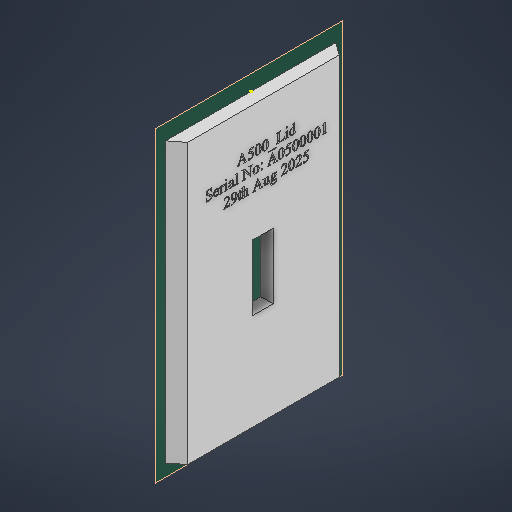
# Autodesk Inventor part: A500_Lid
Saved by Autodesk Inventor 2026.1 (Build 301233000, 233)
## iProperties
Created: 2025-08-29
Part Number: A500_Lid
Material: Generic
Document SubType Name: Modeling
Designer: usman
Density: 1 g/cm^3
Appearance: Default
Author: usman
Autodesk Inventor part; units mm, degrees
(part 1 of 2)
ref_plane "YZ Plane" through (0, 0, 0) normal (1, 0, 0) x (0, 1, 0)
ref_plane "XZ Plane" through (0, 0, 0) normal (0, 1, 0) x (-1, 0, 0)
ref_plane "XY Plane" through (0, 0, 0) normal (0, 0, 1) x (1, 0, 0)
sketch "Sketch1" plane through (0, 0, 0) normal (1, 0, 0) x (0, 1, 0)
  line L0 (-89.45, 54.5) -> (89.45, 54.5)
  line L1 (89.45, 54.5) -> (89.45, -54.5)
  line L2 (89.45, -54.5) -> (-89.45, -54.5)
  line L3 (-89.45, -54.5) -> (-89.45, 54.5)
  line L4 (-89.45, 54.5) -> (89.45, -54.5) construction
  line L5 (89.45, 54.5) -> (-89.45, -54.5) construction
  point P0 (0, 0)
  dimension "d0" = 178.9
  dimension "d1" = 109
  constraints: 12 end point, 2 midpoint, 2 parallel, 1 horizontal, 1 perpendicular
  measures "d0" distance of L0.start L0.end
  measures "d1" distance of L0.end L1.end
extrude "Extrusion1" add sketch "Sketch1" along normal blind 8
sketch "Sketch2" plane through (0, 89.45, 54.5) normal (0, 1, 0) x (1, 0, 0)
  point P0 (0, 54.5)
sketch "Sketch3" plane through (0, 89.45, 54.5) normal (0, 1, 0) x (1, 0, 0)
  line L0 (0, 0) -> (8, 0) projected
  line L1 (0, 0) -> (8, 6.2837)
  line L2 (8, 109) -> (8, 0) projected
  line L3 (0, 109) -> (8, 109) projected
  line L4 (0, 109) -> (8, 103.3983)
  line L5 (0, 109) -> (0, 0) projected
  line L6 (0, 0) -> (8, 0)
  line L7 (0, 109) -> (8, 109)
  line L8 (8, 103.3983) -> (8, 109)
  point P0 (0, 54.5)
  dimension "d4" = 125
  constraints: 10 end point, 3 collinear, 2 point on line
  measures "d4" angle of L5 L4
extrude "Extrusion2" cut sketch "Sketch3" against normal through all contours L1 L2 L0 | L3 L2 L4
sketch "Sketch4" plane through (8, 0, 0) normal (1, 0, 0) x (0, 0, -1)
  line L0 (6.5, 14.45) -> (-6.5, 14.45)
  line L1 (-6.5, 14.45) -> (-6.5, -27.55)
  line L2 (-6.5, -27.55) -> (6.5, -27.55)
  line L3 (6.5, -27.55) -> (6.5, 14.45)
  line L4 (6.5, 14.45) -> (-6.5, -27.55) construction
  line L5 (-6.5, 14.45) -> (6.5, -27.55) construction
  line L6 (48.8983, 89.45) -> (-48.2163, 89.45) projected
  line L7 (-54.5, 89.45) -> (-54.5, -89.45) projected
  point P0 (0, 0)
  point P1 (0, -6.55)
  dimension "d7" = 75
  dimension "d8" = 42
  dimension "d9" = 13
  dimension "d10" = 54.5
  constraints: 12 end point, 2 midpoint, 2 parallel, 1 horizontal, 1 perpendicular
  measures "d7" distance between parallel lines of L0 L6
  measures "d8" distance of L0.end L1.end
  measures "d9" distance of L1.end L2.end
  measures "d10" distance from line of L7 point (0, -6.55)
extrude "Extrusion3" cut sketch "Sketch4" against normal through all
sketch "Sketch6" plane through (8, 0, 0) normal (1, 0, 0) x (0, 0, -1)
  line L0 (-41.7469, 84.5581) -> (46.2409, 84.5581) construction
  line L1 (46.2409, 84.5581) -> (46.2409, 20.4595) construction
  line L2 (46.2409, 20.4595) -> (-41.7469, 20.4595) construction
  line L3 (-41.7469, 20.4595) -> (-41.7469, 84.5581) construction
  line L4 (-12.4626, 61.9812) -> (-14.8333, 61.9812)
  line L5 (-14.8333, 61.9812) -> (-15.2466, 61.025)
  spline S0 degree 2 poles (-15.2466, 61.025) (-15.401, 60.6664) (-15.401, 60.4921) knots 0 0 0 1 1 1
  spline S1 degree 2 poles (-15.401, 60.4921) (-15.401, 60.3526) (-15.1321, 60.1385) (-14.6938, 60.1086) knots 0 0 0 1 2 2 2
  line L6 (-14.6938, 60.1086) -> (-14.6938, 59.9442)
  line L7 (-14.6938, 59.9442) -> (-16.6162, 59.9442)
  line L8 (-16.6162, 59.9442) -> (-16.6162, 60.1086)
  spline S2 degree 2 poles (-16.6162, 60.1086) (-16.2327, 60.1783) (-16.1232, 60.2829) knots 0 0 0 1 1 1
  spline S3 degree 2 poles (-16.1232, 60.2829) (-15.8941, 60.502) (-15.6152, 61.1644) knots 0 0 0 1 1 1
  line L9 (-15.6152, 61.1644) -> (-13.4636, 66.1797)
  line L10 (-13.4636, 66.1797) -> (-13.3043, 66.1797)
  line L11 (-13.3043, 66.1797) -> (-11.1826, 61.1096)
  spline S4 degree 2 poles (-11.1826, 61.1096) (-10.9286, 60.497) (-10.5103, 60.1335) (-10.1367, 60.1086) knots 0 0 0 1 2 2 2
  line L12 (-10.1367, 60.1086) -> (-10.1367, 59.9442)
  line L13 (-10.1367, 59.9442) -> (-12.5423, 59.9442)
  line L14 (-12.5423, 59.9442) -> (-12.5423, 60.1086)
  spline S5 degree 2 poles (-12.5423, 60.1086) (-12.1787, 60.1285) (-11.9197, 60.3327) (-11.9197, 60.4821) knots 0 0 0 1 2 2 2
  spline S6 degree 2 poles (-11.9197, 60.4821) (-11.9197, 60.6813) (-12.099, 61.1096) knots 0 0 0 1 1 1
  line L15 (-12.099, 61.1096) -> (-12.4626, 61.9812)
  line L16 (-12.602, 62.3149) -> (-13.628, 64.7802)
  line L17 (-13.628, 64.7802) -> (-14.6938, 62.3149)
  line L18 (-14.6938, 62.3149) -> (-12.602, 62.3149)
  line L19 (-6.0379, 66.0402) -> (-6.3865, 65.2782)
  line L20 (-6.3865, 65.2782) -> (-8.2193, 65.2782)
  line L21 (-8.2193, 65.2782) -> (-8.6227, 64.4614)
  spline S7 degree 2 poles (-8.6227, 64.4614) (-7.4324, 64.2871) (-6.7351, 63.5749) knots 0 0 0 1 1 1
  spline S8 degree 2 poles (-6.7351, 63.5749) (-6.1375, 62.9623) (-6.1375, 62.1356) knots 0 0 0 1 1 1
  spline S9 degree 2 poles (-6.1375, 62.1356) (-6.1375, 61.6575) (-6.5309, 60.8357) (-7.1236, 60.263) (-7.4872, 60.0886) knots 0 0 0 1 2 3 3 3
  spline S10 degree 2 poles (-7.4872, 60.0886) (-8.0051, 59.8396) (-8.548, 59.8396) knots 0 0 0 1 1 1
  spline S11 degree 2 poles (-8.548, 59.8396) (-9.1008, 59.8396) (-9.5989, 60.2132) (-9.5989, 60.4373) knots 0 0 0 1 2 2 2
  spline S12 degree 2 poles (-9.5989, 60.4373) (-9.5989, 60.5618) (-9.3947, 60.756) (-9.2353, 60.756) knots 0 0 0 1 2 2 2
  spline S13 degree 2 poles (-9.2353, 60.756) (-9.1207, 60.756) (-8.9415, 60.6813) (-8.7323, 60.5319) knots 0 0 0 1 2 2 2
  spline S14 degree 2 poles (-8.7323, 60.5319) (-8.3936, 60.3028) (-8.045, 60.2978) knots 0 0 0 1 1 1
  spline S15 degree 2 poles (-8.045, 60.2978) (-7.522, 60.2978) (-6.7202, 61.0947) (-6.7202, 61.6674) knots 0 0 0 1 2 2 2
  spline S16 degree 2 poles (-6.7202, 61.6674) (-6.7202, 62.2203) (-7.4324, 63.1815) (-8.0599, 63.4405) knots 0 0 0 1 2 2 2
  spline S17 degree 2 poles (-8.0599, 63.4405) (-8.548, 63.6446) (-9.3947, 63.6745) knots 0 0 0 1 1 1
  line L22 (-9.3947, 63.6745) -> (-8.2243, 66.0402)
  line L23 (-8.2243, 66.0402) -> (-6.0379, 66.0402)
  spline S18 degree 2 poles (-5.0966, 62.9574) (-5.0966, 63.9983) (-4.4691, 65.5023) (-3.9461, 65.8709) knots 0 0 0 1 2 2 2
  spline S19 degree 2 poles (-3.9461, 65.8709) (-3.5427, 66.1647) (-3.1094, 66.1647) knots 0 0 0 1 1 1
  spline S20 degree 2 poles (-3.1094, 66.1647) (-2.4072, 66.1647) (-1.8494, 65.4525) knots 0 0 0 1 1 1
  spline S21 degree 2 poles (-1.8494, 65.4525) (-1.1521, 64.566) (-1.1521, 63.052) knots 0 0 0 1 1 1
  spline S22 degree 2 poles (-1.1521, 63.052) (-1.1521, 61.9912) (-1.7647, 60.507) (-2.711, 59.8396) (-3.1542, 59.8396) knots 0 0 0 1 2 3 3 3
  spline S23 degree 2 poles (-3.1542, 59.8396) (-4.0258, 59.8396) (-4.6085, 60.8706) knots 0 0 0 1 1 1
  spline S24 degree 2 poles (-4.6085, 60.8706) (-5.0966, 61.7372) (-5.0966, 62.9574) knots 0 0 0 1 1 1
  spline S25 degree 2 poles (-4.2151, 62.8428) (-4.2151, 61.5877) (-3.9063, 60.7909) knots 0 0 0 1 1 1
  spline S26 degree 2 poles (-3.9063, 60.7909) (-3.6473, 60.1235) (-3.1393, 60.1235) knots 0 0 0 1 1 1
  spline S27 degree 2 poles (-3.1393, 60.1235) (-2.8953, 60.1235) (-2.3773, 60.5568) (-2.2428, 61.0698) knots 0 0 0 1 2 2 2
  spline S28 degree 2 poles (-2.2428, 61.0698) (-2.0336, 61.8417) (-2.0336, 63.2462) knots 0 0 0 1 1 1
  spline S29 degree 2 poles (-2.0336, 63.2462) (-2.0336, 64.2921) (-2.2478, 64.9844) knots 0 0 0 1 1 1
  spline S30 degree 2 poles (-2.2478, 64.9844) (-2.4122, 65.5023) (-2.6662, 65.7165) knots 0 0 0 1 1 1
  spline S31 degree 2 poles (-2.6662, 65.7165) (-2.8504, 65.8659) (-3.1144, 65.8659) knots 0 0 0 1 1 1
  spline S32 degree 2 poles (-3.1144, 65.8659) (-3.4182, 65.8659) (-3.6573, 65.592) knots 0 0 0 1 1 1
  spline S33 degree 2 poles (-3.6573, 65.592) (-3.981, 65.2185) (-4.2151, 63.6197) (-4.2151, 62.8428) knots 0 0 0 1 2 2 2
  spline S34 degree 2 poles (-0.4897, 62.9574) (-0.4897, 63.9983) (0.1378, 65.5023) (0.6607, 65.8709) knots 0 0 0 1 2 2 2
  spline S35 degree 2 poles (0.6607, 65.8709) (1.0642, 66.1647) (1.4975, 66.1647) knots 0 0 0 1 1 1
  spline S36 degree 2 poles (1.4975, 66.1647) (2.1997, 66.1647) (2.7575, 65.4525) knots 0 0 0 1 1 1
  spline S37 degree 2 poles (2.7575, 65.4525) (3.4547, 64.566) (3.4547, 63.052) knots 0 0 0 1 1 1
  spline S38 degree 2 poles (3.4547, 63.052) (3.4547, 61.9912) (2.8422, 60.507) (1.8959, 59.8396) (1.4526, 59.8396) knots 0 0 0 1 2 3 3 3
  spline S39 degree 2 poles (1.4526, 59.8396) (0.5811, 59.8396) (-0.0016, 60.8706) knots 0 0 0 1 1 1
  spline S40 degree 2 poles (-0.0016, 60.8706) (-0.4897, 61.7372) (-0.4897, 62.9574) knots 0 0 0 1 1 1
  spline S41 degree 2 poles (0.3918, 62.8428) (0.3918, 61.5877) (0.7006, 60.7909) knots 0 0 0 1 1 1
  spline S42 degree 2 poles (0.7006, 60.7909) (0.9596, 60.1235) (1.4676, 60.1235) knots 0 0 0 1 1 1
  spline S43 degree 2 poles (1.4676, 60.1235) (1.7116, 60.1235) (2.2296, 60.5568) (2.364, 61.0698) knots 0 0 0 1 2 2 2
  spline S44 degree 2 poles (2.364, 61.0698) (2.5732, 61.8417) (2.5732, 63.2462) knots 0 0 0 1 1 1
  spline S45 degree 2 poles (2.5732, 63.2462) (2.5732, 64.2921) (2.3591, 64.9844) knots 0 0 0 1 1 1
  spline S46 degree 2 poles (2.3591, 64.9844) (2.1947, 65.5023) (1.9407, 65.7165) knots 0 0 0 1 1 1
  spline S47 degree 2 poles (1.9407, 65.7165) (1.7564, 65.8659) (1.4925, 65.8659) knots 0 0 0 1 1 1
  spline S48 degree 2 poles (1.4925, 65.8659) (1.1887, 65.8659) (0.9496, 65.592) knots 0 0 0 1 1 1
  spline S49 degree 2 poles (0.9496, 65.592) (0.6259, 65.2185) (0.3918, 63.6197) (0.3918, 62.8428) knots 0 0 0 1 2 2 2
  line L24 (8.47, 57.962) -> (3.7087, 57.962)
  line L25 (3.7087, 57.962) -> (3.7087, 58.3405)
  line L26 (3.7087, 58.3405) -> (8.47, 58.3405)
  line L27 (8.47, 58.3405) -> (8.47, 57.962)
  line L28 (13.6695, 61.6326) -> (13.8189, 61.6027)
  line L29 (13.8189, 61.6027) -> (13.296, 59.9442)
  line L30 (13.296, 59.9442) -> (8.5796, 59.9442)
  line L31 (8.5796, 59.9442) -> (8.5796, 60.1086)
  line L32 (8.5796, 60.1086) -> (8.8087, 60.1086)
  spline S50 degree 2 poles (8.8087, 60.1086) (9.1922, 60.1086) (9.3565, 60.3626) knots 0 0 0 1 1 1
  spline S51 degree 2 poles (9.3565, 60.3626) (9.4511, 60.502) (9.4511, 61.025) knots 0 0 0 1 1 1
  line L33 (9.4511, 61.025) -> (9.4511, 64.9595)
  spline S52 degree 2 poles (9.4511, 64.9595) (9.4511, 65.5322) (9.3266, 65.6766) knots 0 0 0 1 1 1
  spline S53 degree 2 poles (9.3266, 65.6766) (9.1523, 65.8759) (8.8087, 65.8759) knots 0 0 0 1 1 1
  line L34 (8.8087, 65.8759) -> (8.5796, 65.8759)
  line L35 (8.5796, 65.8759) -> (8.5796, 66.0402)
  line L36 (8.5796, 66.0402) -> (11.3337, 66.0402)
  line L37 (11.3337, 66.0402) -> (11.3337, 65.8759)
  spline S54 degree 2 poles (11.3337, 65.8759) (10.8456, 65.8808) (10.4572, 65.6916) (10.3127, 65.4027) (10.3127, 64.8599) knots 0 0 0 1 2 3 3 3
  line L38 (10.3127, 64.8599) -> (10.3127, 61.0299)
  spline S55 degree 2 poles (10.3127, 61.0299) (10.3127, 60.6564) (10.3825, 60.517) knots 0 0 0 1 1 1
  spline S56 degree 2 poles (10.3825, 60.517) (10.4373, 60.4223) (10.6614, 60.3327) (11.254, 60.3327) knots 0 0 0 1 2 2 2
  line L39 (11.254, 60.3327) -> (11.6973, 60.3327)
  spline S57 degree 2 poles (11.6973, 60.3327) (12.3995, 60.3327) (12.9673, 60.5419) (13.4355, 61.0648) (13.6695, 61.6326) knots 0 0 0 1 2 3 3 3
  line L40 (15.7215, 64.1825) -> (15.7215, 60.8755)
  spline S58 degree 2 poles (15.7215, 60.8755) (15.7215, 60.4921) (15.831, 60.2331) (16.0551, 60.1086) (16.344, 60.1086) knots 0 0 0 1 2 3 3 3
  line L41 (16.344, 60.1086) -> (16.344, 59.9442)
  line L42 (16.344, 59.9442) -> (14.3469, 59.9442)
  line L43 (14.3469, 59.9442) -> (14.3469, 60.1086)
  spline S59 degree 2 poles (14.3469, 60.1086) (14.6457, 60.1086) (14.8549, 60.2231) (14.9744, 60.4921) (14.9744, 60.8755) knots 0 0 0 1 2 3 3 3
  line L44 (14.9744, 60.8755) -> (14.9744, 62.4593)
  spline S60 degree 2 poles (14.9744, 62.4593) (14.9744, 63.1267) (14.9345, 63.3259) knots 0 0 0 1 1 1
  spline S61 degree 2 poles (14.9345, 63.3259) (14.9047, 63.4703) (14.7652, 63.5849) (14.6507, 63.5849) knots 0 0 0 1 2 2 2
  spline S62 degree 2 poles (14.6507, 63.5849) (14.5262, 63.5849) (14.3469, 63.5152) knots 0 0 0 1 1 1
  line L45 (14.3469, 63.5152) -> (14.2821, 63.6795)
  line L46 (14.2821, 63.6795) -> (15.5222, 64.1825)
  line L47 (15.5222, 64.1825) -> (15.7215, 64.1825)
  spline S63 degree 2 poles (15.3479, 66.339) (15.5372, 66.339) (15.8011, 66.0751) (15.8011, 65.8858) knots 0 0 0 1 2 2 2
  spline S64 degree 2 poles (15.8011, 65.8858) (15.8011, 65.6966) (15.5372, 65.4276) (15.3479, 65.4276) knots 0 0 0 1 2 2 2
  spline S65 degree 2 poles (15.3479, 65.4276) (15.1587, 65.4276) (14.8897, 65.6966) (14.8897, 65.8858) knots 0 0 0 1 2 2 2
  spline S66 degree 2 poles (14.8897, 65.8858) (14.8897, 66.0751) (15.1537, 66.339) (15.3479, 66.339) knots 0 0 0 1 2 2 2
  spline S67 degree 2 poles (19.7655, 60.4074) (19.4667, 60.0936) (18.889, 59.8197) (18.5553, 59.8197) knots 0 0 0 1 2 2 2
  spline S68 degree 2 poles (18.5553, 59.8197) (17.8829, 59.8197) (16.8769, 60.9453) (16.8769, 61.8318) knots 0 0 0 1 2 2 2
  spline S69 degree 2 poles (16.8769, 61.8318) (16.8769, 62.7133) (17.9925, 64.1825) (18.8691, 64.1825) knots 0 0 0 1 2 2 2
  spline S70 degree 2 poles (18.8691, 64.1825) (19.4119, 64.1825) (19.7655, 63.8339) knots 0 0 0 1 1 1
  line L48 (19.7655, 63.8339) -> (19.7655, 64.6059)
  spline S71 degree 2 poles (19.7655, 64.6059) (19.7655, 65.3081) (19.6958, 65.6268) (19.5564, 65.7414) (19.4468, 65.7414) knots 0 0 0 1 2 3 3 3
  spline S72 degree 2 poles (19.4468, 65.7414) (19.3322, 65.7414) (19.138, 65.6717) knots 0 0 0 1 1 1
  line L49 (19.138, 65.6717) -> (19.0782, 65.836)
  line L50 (19.0782, 65.836) -> (20.3034, 66.339)
  line L51 (20.3034, 66.339) -> (20.5076, 66.339)
  line L52 (20.5076, 66.339) -> (20.5076, 61.5728)
  spline S73 degree 2 poles (20.5076, 61.5728) (20.5076, 60.8556) (20.5773, 60.5369) (20.7218, 60.4124) (20.8214, 60.4124) knots 0 0 0 1 2 3 3 3
  spline S74 degree 2 poles (20.8214, 60.4124) (20.9409, 60.4124) (21.1451, 60.4871) knots 0 0 0 1 1 1
  line L53 (21.1451, 60.4871) -> (21.1949, 60.3227)
  line L54 (21.1949, 60.3227) -> (19.9747, 59.8197)
  line L55 (19.9747, 59.8197) -> (19.7655, 59.8197)
  line L56 (19.7655, 59.8197) -> (19.7655, 60.4074)
  line L57 (19.7655, 60.7261) -> (19.7655, 62.8378)
  spline S75 degree 2 poles (19.7655, 62.8378) (19.7406, 63.1466) (19.4667, 63.6496) (19.0235, 63.9036) (18.8143, 63.9036) knots 0 0 0 1 2 3 3 3
  spline S76 degree 2 poles (18.8143, 63.9036) (18.4158, 63.9036) (18.1071, 63.55) knots 0 0 0 1 1 1
  spline S77 degree 2 poles (18.1071, 63.55) (17.6987, 63.0819) (17.6987, 62.1854) knots 0 0 0 1 1 1
  spline S78 degree 2 poles (17.6987, 62.1854) (17.6987, 61.279) (18.4905, 60.3128) (18.9736, 60.3128) knots 0 0 0 1 2 2 2
  spline S79 degree 2 poles (18.9736, 60.3128) (19.382, 60.3128) (19.7655, 60.7261) knots 0 0 0 1 1 1
  line L58 (-32.9196, 56.538) -> (-32.9196, 54.4313)
  line L59 (-32.9196, 54.4313) -> (-33.0839, 54.4313)
  spline S80 degree 2 poles (-33.0839, 54.4313) (-33.1636, 55.0389) (-33.5869, 55.7561) (-34.3589, 56.1794) (-34.7772, 56.1794) knots 0 0 0 1 2 3 3 3
  spline S81 degree 2 poles (-34.7772, 56.1794) (-35.2454, 56.1794) (-35.858, 55.6066) (-35.858, 55.2431) knots 0 0 0 1 2 2 2
  spline S82 degree 2 poles (-35.858, 55.2431) (-35.858, 54.9642) (-35.6637, 54.7351) knots 0 0 0 1 1 1
  spline S83 degree 2 poles (-35.6637, 54.7351) (-35.3848, 54.3964) (-34.334, 53.8336) knots 0 0 0 1 1 1
  spline S84 degree 2 poles (-34.334, 53.8336) (-33.4823, 53.3754) (-32.8548, 52.8873) (-32.5161, 52.22) (-32.5161, 51.8564) knots 0 0 0 1 2 3 3 3
  spline S85 degree 2 poles (-32.5161, 51.8564) (-32.5161, 51.1641) (-33.5919, 50.1631) (-34.4386, 50.1631) knots 0 0 0 1 2 2 2
  spline S86 degree 2 poles (-34.4386, 50.1631) (-34.7025, 50.1631) (-34.9366, 50.2029) knots 0 0 0 1 1 1
  spline S87 degree 2 poles (-34.9366, 50.2029) (-35.0761, 50.2278) (-35.9526, 50.5117) (-36.0721, 50.5117) knots 0 0 0 1 2 2 2
  spline S88 degree 2 poles (-36.0721, 50.5117) (-36.1817, 50.5117) (-36.3162, 50.3772) (-36.3461, 50.1631) knots 0 0 0 1 2 2 2
  line L60 (-36.3461, 50.1631) -> (-36.5104, 50.1631)
  line L61 (-36.5104, 50.1631) -> (-36.5104, 52.2548)
  line L62 (-36.5104, 52.2548) -> (-36.3461, 52.2548)
  spline S89 degree 2 poles (-36.3461, 52.2548) (-36.2315, 51.5974) (-35.8331, 50.945) (-35.0163, 50.5117) (-34.5332, 50.5117) knots 0 0 0 1 2 3 3 3
  spline S90 degree 2 poles (-34.5332, 50.5117) (-33.9704, 50.5117) (-33.318, 51.1044) (-33.318, 51.5128) knots 0 0 0 1 2 2 2
  spline S91 degree 2 poles (-33.318, 51.5128) (-33.318, 51.7369) (-33.567, 52.1951) (-33.826, 52.3943) knots 0 0 0 1 2 2 2
  spline S92 degree 2 poles (-33.826, 52.3943) (-34.0003, 52.5288) (-35.5691, 53.4053) (-36.2315, 53.9282) (-36.5752, 54.5558) (-36.5752, 54.9343) knots 0 0 0 1 2 3 4 4 4
  spline S93 degree 2 poles (-36.5752, 54.9343) (-36.5752, 55.5917) (-35.5641, 56.538) (-34.7822, 56.538) knots 0 0 0 1 2 2 2
  spline S94 degree 2 poles (-34.7822, 56.538) (-34.2991, 56.538) (-33.7513, 56.2989) knots 0 0 0 1 1 1
  spline S95 degree 2 poles (-33.7513, 56.2989) (-33.4973, 56.1893) (-33.3927, 56.1893) knots 0 0 0 1 1 1
  spline S96 degree 2 poles (-33.3927, 56.1893) (-33.2781, 56.1893) (-33.1287, 56.3288) (-33.0839, 56.538) knots 0 0 0 1 2 2 2
  line L63 (-33.0839, 56.538) -> (-32.9196, 56.538)
  spline S97 degree 2 poles (-31.0519, 52.8674) (-31.0569, 51.951) (-30.6086, 51.4331) knots 0 0 0 1 1 1
  spline S98 degree 2 poles (-30.6086, 51.4331) (-30.1554, 50.9101) (-29.5478, 50.9101) knots 0 0 0 1 1 1
  spline S99 degree 2 poles (-29.5478, 50.9101) (-29.1444, 50.9101) (-28.5468, 51.3534) (-28.3426, 51.8962) knots 0 0 0 1 2 2 2
  line L64 (-28.3426, 51.8962) -> (-28.2031, 51.8066)
  spline S100 degree 2 poles (-28.2031, 51.8066) (-28.2977, 51.189) (-29.2042, 50.178) (-29.8915, 50.178) knots 0 0 0 1 2 2 2
  spline S101 degree 2 poles (-29.8915, 50.178) (-30.6336, 50.178) (-31.6894, 51.3335) (-31.6894, 52.3046) knots 0 0 0 1 2 2 2
  spline S102 degree 2 poles (-31.6894, 52.3046) (-31.6894, 53.3605) (-30.6037, 54.5408) (-29.7869, 54.5408) knots 0 0 0 1 2 2 2
  spline S103 degree 2 poles (-29.7869, 54.5408) (-29.0946, 54.5408) (-28.2031, 53.6294) (-28.2031, 52.8674) knots 0 0 0 1 2 2 2
  line L65 (-28.2031, 52.8674) -> (-31.0519, 52.8674)
  line L66 (-31.0519, 53.1264) -> (-29.1394, 53.1264)
  spline S104 degree 2 poles (-29.1394, 53.1264) (-29.1643, 53.5199) (-29.2341, 53.6842) knots 0 0 0 1 1 1
  spline S105 degree 2 poles (-29.2341, 53.6842) (-29.3486, 53.9332) (-29.7919, 54.2221) (-30.0359, 54.2221) knots 0 0 0 1 2 2 2
  spline S106 degree 2 poles (-30.0359, 54.2221) (-30.4094, 54.2221) (-31.0021, 53.6444) (-31.0519, 53.1264) knots 0 0 0 1 2 2 2
  line L67 (-26.445, 54.5408) -> (-26.445, 53.6145)
  spline S107 degree 2 poles (-26.445, 53.6145) (-25.9271, 54.5408) (-25.3842, 54.5408) knots 0 0 0 1 1 1
  spline S108 degree 2 poles (-25.3842, 54.5408) (-25.1402, 54.5408) (-24.8165, 54.242) (-24.8165, 54.0428) knots 0 0 0 1 2 2 2
  spline S109 degree 2 poles (-24.8165, 54.0428) (-24.8165, 53.8685) (-25.0505, 53.6244) (-25.2099, 53.6244) knots 0 0 0 1 2 2 2
  spline S110 degree 2 poles (-25.2099, 53.6244) (-25.3693, 53.6244) (-25.7577, 53.9332) (-25.8524, 53.9332) knots 0 0 0 1 2 2 2
  spline S111 degree 2 poles (-25.8524, 53.9332) (-25.9321, 53.9332) (-26.0267, 53.8436) knots 0 0 0 1 1 1
  spline S112 degree 2 poles (-26.0267, 53.8436) (-26.2309, 53.6593) (-26.445, 53.236) knots 0 0 0 1 1 1
  line L68 (-26.445, 53.236) -> (-26.445, 51.2637)
  spline S113 degree 2 poles (-26.445, 51.2637) (-26.445, 50.9201) (-26.3604, 50.7458) knots 0 0 0 1 1 1
  spline S114 degree 2 poles (-26.3604, 50.7458) (-26.3006, 50.6262) (-26.0068, 50.4669) (-25.7279, 50.4669) knots 0 0 0 1 2 2 2
  line L69 (-25.7279, 50.4669) -> (-25.7279, 50.3025)
  line L70 (-25.7279, 50.3025) -> (-27.8396, 50.3025)
  line L71 (-27.8396, 50.3025) -> (-27.8396, 50.4669)
  spline S115 degree 2 poles (-27.8396, 50.4669) (-27.5258, 50.4669) (-27.3714, 50.5665) knots 0 0 0 1 1 1
  spline S116 degree 2 poles (-27.3714, 50.5665) (-27.2618, 50.6362) (-27.217, 50.7956) knots 0 0 0 1 1 1
  spline S117 degree 2 poles (-27.217, 50.7956) (-27.1921, 50.8753) (-27.1921, 51.2339) knots 0 0 0 1 1 1
  line L72 (-27.1921, 51.2339) -> (-27.1921, 52.8226)
  spline S118 degree 2 poles (-27.1921, 52.8226) (-27.1921, 53.5398) (-27.2519, 53.8137) (-27.4063, 53.9432) (-27.5258, 53.9432) knots 0 0 0 1 2 3 3 3
  spline S119 degree 2 poles (-27.5258, 53.9432) (-27.6652, 53.9432) (-27.8396, 53.8735) knots 0 0 0 1 1 1
  line L73 (-27.8396, 53.8735) -> (-27.8844, 54.0378)
  line L74 (-27.8844, 54.0378) -> (-26.6343, 54.5408)
  line L75 (-26.6343, 54.5408) -> (-26.445, 54.5408)
  line L76 (-23.1679, 54.5408) -> (-23.1679, 51.2339)
  spline S120 degree 2 poles (-23.1679, 51.2339) (-23.1679, 50.8504) (-23.0584, 50.5914) (-22.8343, 50.4669) (-22.5454, 50.4669) knots 0 0 0 1 2 3 3 3
  line L77 (-22.5454, 50.4669) -> (-22.5454, 50.3025)
  line L78 (-22.5454, 50.3025) -> (-24.5425, 50.3025)
  line L79 (-24.5425, 50.3025) -> (-24.5425, 50.4669)
  spline S121 degree 2 poles (-24.5425, 50.4669) (-24.2437, 50.4669) (-24.0345, 50.5814) (-23.915, 50.8504) (-23.915, 51.2339) knots 0 0 0 1 2 3 3 3
  line L80 (-23.915, 51.2339) -> (-23.915, 52.8176)
  spline S122 degree 2 poles (-23.915, 52.8176) (-23.915, 53.485) (-23.9548, 53.6842) knots 0 0 0 1 1 1
  spline S123 degree 2 poles (-23.9548, 53.6842) (-23.9847, 53.8286) (-24.1242, 53.9432) (-24.2387, 53.9432) knots 0 0 0 1 2 2 2
  spline S124 degree 2 poles (-24.2387, 53.9432) (-24.3632, 53.9432) (-24.5425, 53.8735) knots 0 0 0 1 1 1
  line L81 (-24.5425, 53.8735) -> (-24.6073, 54.0378)
  line L82 (-24.6073, 54.0378) -> (-23.3672, 54.5408)
  line L83 (-23.3672, 54.5408) -> (-23.1679, 54.5408)
  spline S125 degree 2 poles (-23.5415, 56.6973) (-23.3522, 56.6973) (-23.0883, 56.4334) (-23.0883, 56.2441) knots 0 0 0 1 2 2 2
  spline S126 degree 2 poles (-23.0883, 56.2441) (-23.0883, 56.0549) (-23.3522, 55.7859) (-23.5415, 55.7859) knots 0 0 0 1 2 2 2
  spline S127 degree 2 poles (-23.5415, 55.7859) (-23.7307, 55.7859) (-23.9997, 56.0549) (-23.9997, 56.2441) knots 0 0 0 1 2 2 2
  spline S128 degree 2 poles (-23.9997, 56.2441) (-23.9997, 56.4334) (-23.7357, 56.6973) (-23.5415, 56.6973) knots 0 0 0 1 2 2 2
  spline S129 degree 2 poles (-19.6966, 50.9002) (-20.3291, 50.4071) (-20.4935, 50.3324) knots 0 0 0 1 1 1
  spline S130 degree 2 poles (-20.4935, 50.3324) (-20.7325, 50.2179) (-21.0065, 50.2179) knots 0 0 0 1 1 1
  spline S131 degree 2 poles (-21.0065, 50.2179) (-21.4348, 50.2179) (-21.9876, 50.8006) (-21.9876, 51.2787) knots 0 0 0 1 2 2 2
  spline S132 degree 2 poles (-21.9876, 51.2787) (-21.9876, 51.5775) (-21.8531, 51.8016) knots 0 0 0 1 1 1
  spline S133 degree 2 poles (-21.8531, 51.8016) (-21.6688, 52.1054) (-20.7574, 52.6433) (-19.6966, 53.0318) knots 0 0 0 1 2 2 2
  line L84 (-19.6966, 53.0318) -> (-19.6966, 53.1911)
  spline S134 degree 2 poles (-19.6966, 53.1911) (-19.6966, 53.8087) (-20.0851, 54.2669) (-20.4586, 54.2669) knots 0 0 0 1 2 2 2
  spline S135 degree 2 poles (-20.4586, 54.2669) (-20.7375, 54.2669) (-20.9068, 54.1125) knots 0 0 0 1 1 1
  spline S136 degree 2 poles (-20.9068, 54.1125) (-21.0762, 53.9631) (-21.0762, 53.7639) knots 0 0 0 1 1 1
  line L85 (-21.0762, 53.7639) -> (-21.0662, 53.5049)
  spline S137 degree 2 poles (-21.0662, 53.5049) (-21.0662, 53.2957) (-21.2804, 53.0716) (-21.4497, 53.0716) knots 0 0 0 1 2 2 2
  spline S138 degree 2 poles (-21.4497, 53.0716) (-21.6141, 53.0716) (-21.8282, 53.3057) (-21.8282, 53.5099) knots 0 0 0 1 2 2 2
  spline S139 degree 2 poles (-21.8282, 53.5099) (-21.8282, 53.8934) (-21.0363, 54.5408) (-20.3241, 54.5408) knots 0 0 0 1 2 2 2
  spline S140 degree 2 poles (-20.3241, 54.5408) (-19.7763, 54.5408) (-19.4277, 54.3566) knots 0 0 0 1 1 1
  spline S141 degree 2 poles (-19.4277, 54.3566) (-19.1587, 54.2171) (-19.0342, 53.9233) knots 0 0 0 1 1 1
  spline S142 degree 2 poles (-19.0342, 53.9233) (-18.9545, 53.729) (-18.9545, 53.1314) knots 0 0 0 1 1 1
  line L86 (-18.9545, 53.1314) -> (-18.9545, 51.7319)
  spline S143 degree 2 poles (-18.9545, 51.7319) (-18.9545, 51.1442) (-18.9097, 50.8802) (-18.8051, 50.7906) (-18.7404, 50.7906) knots 0 0 0 1 2 3 3 3
  spline S144 degree 2 poles (-18.7404, 50.7906) (-18.6657, 50.7906) (-18.6109, 50.8205) knots 0 0 0 1 1 1
  spline S145 degree 2 poles (-18.6109, 50.8205) (-18.5163, 50.8802) (-18.2473, 51.1492) knots 0 0 0 1 1 1
  line L87 (-18.2473, 51.1492) -> (-18.2473, 50.9002)
  spline S146 degree 2 poles (-18.2473, 50.9002) (-18.7503, 50.2228) (-19.2085, 50.2228) knots 0 0 0 1 1 1
  spline S147 degree 2 poles (-19.2085, 50.2228) (-19.4326, 50.2228) (-19.6916, 50.5266) (-19.6966, 50.9002) knots 0 0 0 1 2 2 2
  line L88 (-19.6966, 51.189) -> (-19.6966, 52.7579)
  spline S148 degree 2 poles (-19.6966, 52.7579) (-20.3739, 52.4889) (-20.5732, 52.3744) knots 0 0 0 1 1 1
  spline S149 degree 2 poles (-20.5732, 52.3744) (-20.9268, 52.1801) (-21.2306, 51.7468) (-21.2306, 51.4928) knots 0 0 0 1 2 2 2
  spline S150 degree 2 poles (-21.2306, 51.4928) (-21.2306, 51.1691) (-20.8471, 50.7408) (-20.5931, 50.7408) knots 0 0 0 1 2 2 2
  spline S151 degree 2 poles (-20.5931, 50.7408) (-20.2544, 50.7408) (-19.6966, 51.189) knots 0 0 0 1 1 1
  line L89 (-16.5191, 56.6973) -> (-16.5191, 51.2339)
  spline S152 degree 2 poles (-16.5191, 51.2339) (-16.5191, 50.8504) (-16.4046, 50.5964) (-16.1705, 50.4669) (-15.8517, 50.4669) knots 0 0 0 1 2 3 3 3
  line L90 (-15.8517, 50.4669) -> (-15.8517, 50.3025)
  line L91 (-15.8517, 50.3025) -> (-17.8788, 50.3025)
  line L92 (-17.8788, 50.3025) -> (-17.8788, 50.4669)
  spline S153 degree 2 poles (-17.8788, 50.4669) (-17.5949, 50.4669) (-17.3857, 50.5814) (-17.2662, 50.8504) (-17.2662, 51.2339) knots 0 0 0 1 2 3 3 3
  line L93 (-17.2662, 51.2339) -> (-17.2662, 54.9741)
  spline S154 degree 2 poles (-17.2662, 54.9741) (-17.2662, 55.6664) (-17.3309, 55.9851) (-17.4704, 56.0997) (-17.575, 56.0997) knots 0 0 0 1 2 3 3 3
  spline S155 degree 2 poles (-17.575, 56.0997) (-17.6945, 56.0997) (-17.8738, 56.03) knots 0 0 0 1 1 1
  line L94 (-17.8738, 56.03) -> (-17.9485, 56.1943)
  line L95 (-17.9485, 56.1943) -> (-16.7233, 56.6973)
  line L96 (-16.7233, 56.6973) -> (-16.5191, 56.6973)
  line L97 (-13.4861, 56.3985) -> (-11.8425, 56.3985)
  line L98 (-11.8425, 56.3985) -> (-8.1072, 51.8215)
  line L99 (-8.1072, 51.8215) -> (-8.1072, 55.3427)
  spline S156 degree 2 poles (-8.1072, 55.3427) (-8.1072, 55.9055) (-8.2317, 56.0449) knots 0 0 0 1 1 1
  spline S157 degree 2 poles (-8.2317, 56.0449) (-8.4011, 56.2342) (-8.7597, 56.2342) knots 0 0 0 1 1 1
  line L100 (-8.7597, 56.2342) -> (-8.9688, 56.2342)
  line L101 (-8.9688, 56.2342) -> (-8.9688, 56.3985)
  line L102 (-8.9688, 56.3985) -> (-6.8522, 56.3985)
  line L103 (-6.8522, 56.3985) -> (-6.8522, 56.2342)
  line L104 (-6.8522, 56.2342) -> (-7.0663, 56.2342)
  spline S158 degree 2 poles (-7.0663, 56.2342) (-7.4548, 56.2342) (-7.6142, 56.0001) knots 0 0 0 1 1 1
  spline S159 degree 2 poles (-7.6142, 56.0001) (-7.7138, 55.8557) (-7.7138, 55.3427) knots 0 0 0 1 1 1
  line L105 (-7.7138, 55.3427) -> (-7.7138, 50.2029)
  line L106 (-7.7138, 50.2029) -> (-7.8732, 50.2029)
  line L107 (-7.8732, 50.2029) -> (-11.8923, 55.1136)
  line L108 (-11.8923, 55.1136) -> (-11.8923, 51.3584)
  spline S160 degree 2 poles (-11.8923, 51.3584) (-11.8923, 50.7956) (-11.7728, 50.6561) knots 0 0 0 1 1 1
  spline S161 degree 2 poles (-11.7728, 50.6561) (-11.5985, 50.4669) (-11.2449, 50.4669) knots 0 0 0 1 1 1
  line L109 (-11.2449, 50.4669) -> (-11.0307, 50.4669)
  line L110 (-11.0307, 50.4669) -> (-11.0307, 50.3025)
  line L111 (-11.0307, 50.3025) -> (-13.1474, 50.3025)
  line L112 (-13.1474, 50.3025) -> (-13.1474, 50.4669)
  line L113 (-13.1474, 50.4669) -> (-12.9382, 50.4669)
  spline S162 degree 2 poles (-12.9382, 50.4669) (-12.5448, 50.4669) (-12.3854, 50.701) knots 0 0 0 1 1 1
  spline S163 degree 2 poles (-12.3854, 50.701) (-12.2858, 50.8454) (-12.2858, 51.3584) knots 0 0 0 1 1 1
  line L114 (-12.2858, 51.3584) -> (-12.2858, 55.5967)
  spline S164 degree 2 poles (-12.2858, 55.5967) (-12.5497, 55.9104) (-12.8237, 56.1097) (-13.0926, 56.1943) knots 0 0 0 1 2 2 2
  spline S165 degree 2 poles (-13.0926, 56.1943) (-13.2221, 56.2342) (-13.4861, 56.2342) knots 0 0 0 1 1 1
  line L115 (-13.4861, 56.2342) -> (-13.4861, 56.3985)
  spline S166 degree 2 poles (-4.4168, 54.5408) (-3.4805, 54.5408) (-2.9177, 53.8286) knots 0 0 0 1 1 1
  spline S167 degree 2 poles (-2.9177, 53.8286) (-2.4346, 53.226) (-2.4346, 52.4391) knots 0 0 0 1 1 1
  spline S168 degree 2 poles (-2.4346, 52.4391) (-2.4346, 51.8863) (-2.9675, 50.7508) (-3.8938, 50.178) (-4.4666, 50.178) knots 0 0 0 1 2 3 3 3
  spline S169 degree 2 poles (-4.4666, 50.178) (-5.3979, 50.178) (-5.9457, 50.9201) knots 0 0 0 1 1 1
  spline S170 degree 2 poles (-5.9457, 50.9201) (-6.4089, 51.5426) (-6.4089, 52.3196) knots 0 0 0 1 1 1
  spline S171 degree 2 poles (-6.4089, 52.3196) (-6.4089, 52.8873) (-5.8461, 54.0079) (-4.9297, 54.5408) (-4.4168, 54.5408) knots 0 0 0 1 2 3 3 3
  spline S172 degree 2 poles (-4.5562, 54.247) (-4.7953, 54.247) (-5.2734, 53.9631) (-5.5722, 53.2559) (-5.5722, 52.6981) knots 0 0 0 1 2 3 3 3
  spline S173 degree 2 poles (-5.5722, 52.6981) (-5.5722, 51.8016) (-4.86, 50.4968) (-4.2723, 50.4968) knots 0 0 0 1 2 2 2
  spline S174 degree 2 poles (-4.2723, 50.4968) (-3.839, 50.4968) (-3.2713, 51.2139) (-3.2713, 52.0905) knots 0 0 0 1 2 2 2
  spline S175 degree 2 poles (-3.2713, 52.0905) (-3.2713, 53.1862) (-3.7444, 53.8137) knots 0 0 0 1 1 1
  spline S176 degree 2 poles (-3.7444, 53.8137) (-4.0632, 54.247) (-4.5562, 54.247) knots 0 0 0 1 1 1
  spline S177 degree 2 poles (-0.8209, 51.1741) (-0.6117, 51.1741) (-0.3229, 50.8802) (-0.3229, 50.6761) knots 0 0 0 1 2 2 2
  spline S178 degree 2 poles (-0.3229, 50.6761) (-0.3229, 50.4669) (-0.6167, 50.178) (-0.8209, 50.178) knots 0 0 0 1 2 2 2
  spline S179 degree 2 poles (-0.8209, 50.178) (-1.0301, 50.178) (-1.319, 50.4669) (-1.319, 50.6761) knots 0 0 0 1 2 2 2
  spline S180 degree 2 poles (-1.319, 50.6761) (-1.319, 50.8802) (-1.0301, 51.1741) (-0.8209, 51.1741) knots 0 0 0 1 2 2 2
  spline S181 degree 2 poles (-0.811, 54.5408) (-0.6068, 54.5408) (-0.3129, 54.247) (-0.3129, 54.0428) knots 0 0 0 1 2 2 2
  spline S182 degree 2 poles (-0.3129, 54.0428) (-0.3129, 53.8386) (-0.6068, 53.5448) (-0.811, 53.5448) knots 0 0 0 1 2 2 2
  spline S183 degree 2 poles (-0.811, 53.5448) (-1.0152, 53.5448) (-1.309, 53.8386) (-1.309, 54.0428) knots 0 0 0 1 2 2 2
  spline S184 degree 2 poles (-1.309, 54.0428) (-1.309, 54.247) (-1.0152, 54.5408) (-0.811, 54.5408) knots 0 0 0 1 2 2 2
  line L116 (6.9734, 52.3395) -> (4.6027, 52.3395)
  line L117 (4.6027, 52.3395) -> (4.1894, 51.3833)
  spline S185 degree 2 poles (4.1894, 51.3833) (4.035, 51.0247) (4.035, 50.8504) knots 0 0 0 1 1 1
  spline S186 degree 2 poles (4.035, 50.8504) (4.035, 50.7109) (4.3039, 50.4968) (4.7422, 50.4669) knots 0 0 0 1 2 2 2
  line L118 (4.7422, 50.4669) -> (4.7422, 50.3025)
  line L119 (4.7422, 50.3025) -> (2.8197, 50.3025)
  line L120 (2.8197, 50.3025) -> (2.8197, 50.4669)
  spline S187 degree 2 poles (2.8197, 50.4669) (3.2032, 50.5366) (3.3128, 50.6412) knots 0 0 0 1 1 1
  spline S188 degree 2 poles (3.3128, 50.6412) (3.5419, 50.8603) (3.8208, 51.5227) knots 0 0 0 1 1 1
  line L121 (3.8208, 51.5227) -> (5.9723, 56.538)
  line L122 (5.9723, 56.538) -> (6.1317, 56.538)
  line L123 (6.1317, 56.538) -> (8.2534, 51.4679)
  spline S189 degree 2 poles (8.2534, 51.4679) (8.5074, 50.8553) (8.9257, 50.4918) (9.2992, 50.4669) knots 0 0 0 1 2 2 2
  line L124 (9.2992, 50.4669) -> (9.2992, 50.3025)
  line L125 (9.2992, 50.3025) -> (6.8937, 50.3025)
  line L126 (6.8937, 50.3025) -> (6.8937, 50.4669)
  spline S190 degree 2 poles (6.8937, 50.4669) (7.2573, 50.4868) (7.5163, 50.691) (7.5163, 50.8404) knots 0 0 0 1 2 2 2
  spline S191 degree 2 poles (7.5163, 50.8404) (7.5163, 51.0396) (7.337, 51.4679) knots 0 0 0 1 1 1
  line L127 (7.337, 51.4679) -> (6.9734, 52.3395)
  line L128 (6.8339, 52.6732) -> (5.808, 55.1385)
  line L129 (5.808, 55.1385) -> (4.7422, 52.6732)
  line L130 (4.7422, 52.6732) -> (6.8339, 52.6732)
  spline S192 degree 2 poles (9.7325, 53.3157) (9.7325, 54.3566) (10.3601, 55.8606) (10.883, 56.2292) knots 0 0 0 1 2 2 2
  spline S193 degree 2 poles (10.883, 56.2292) (11.2864, 56.523) (11.7197, 56.523) knots 0 0 0 1 1 1
  spline S194 degree 2 poles (11.7197, 56.523) (12.4219, 56.523) (12.9797, 55.8108) knots 0 0 0 1 1 1
  spline S195 degree 2 poles (12.9797, 55.8108) (13.677, 54.9243) (13.677, 53.4103) knots 0 0 0 1 1 1
  spline S196 degree 2 poles (13.677, 53.4103) (13.677, 52.3495) (13.0644, 50.8653) (12.1181, 50.1979) (11.6749, 50.1979) knots 0 0 0 1 2 3 3 3
  spline S197 degree 2 poles (11.6749, 50.1979) (10.8033, 50.1979) (10.2206, 51.2289) knots 0 0 0 1 1 1
  spline S198 degree 2 poles (10.2206, 51.2289) (9.7325, 52.0955) (9.7325, 53.3157) knots 0 0 0 1 1 1
  spline S199 degree 2 poles (10.6141, 53.2011) (10.6141, 51.9461) (10.9228, 51.1492) knots 0 0 0 1 1 1
  spline S200 degree 2 poles (10.9228, 51.1492) (11.1818, 50.4818) (11.6898, 50.4818) knots 0 0 0 1 1 1
  spline S201 degree 2 poles (11.6898, 50.4818) (11.9339, 50.4818) (12.4518, 50.9151) (12.5863, 51.4281) knots 0 0 0 1 2 2 2
  spline S202 degree 2 poles (12.5863, 51.4281) (12.7955, 52.2001) (12.7955, 53.6045) knots 0 0 0 1 1 1
  spline S203 degree 2 poles (12.7955, 53.6045) (12.7955, 54.6504) (12.5813, 55.3427) knots 0 0 0 1 1 1
  spline S204 degree 2 poles (12.5813, 55.3427) (12.417, 55.8606) (12.163, 56.0748) knots 0 0 0 1 1 1
  spline S205 degree 2 poles (12.163, 56.0748) (11.9787, 56.2242) (11.7147, 56.2242) knots 0 0 0 1 1 1
  spline S206 degree 2 poles (11.7147, 56.2242) (11.4109, 56.2242) (11.1719, 55.9503) knots 0 0 0 1 1 1
  spline S207 degree 2 poles (11.1719, 55.9503) (10.8481, 55.5768) (10.6141, 53.9781) (10.6141, 53.2011) knots 0 0 0 1 2 2 2
  line L131 (18.005, 56.3985) -> (17.6563, 55.6365)
  line L132 (17.6563, 55.6365) -> (15.8235, 55.6365)
  line L133 (15.8235, 55.6365) -> (15.4201, 54.8197)
  spline S208 degree 2 poles (15.4201, 54.8197) (16.6104, 54.6454) (17.3077, 53.9332) knots 0 0 0 1 1 1
  spline S209 degree 2 poles (17.3077, 53.9332) (17.9054, 53.3206) (17.9054, 52.4939) knots 0 0 0 1 1 1
  spline S210 degree 2 poles (17.9054, 52.4939) (17.9054, 52.0158) (17.5119, 51.194) (16.9192, 50.6213) (16.5557, 50.447) knots 0 0 0 1 2 3 3 3
  spline S211 degree 2 poles (16.5557, 50.447) (16.0377, 50.1979) (15.4948, 50.1979) knots 0 0 0 1 1 1
  spline S212 degree 2 poles (15.4948, 50.1979) (14.942, 50.1979) (14.444, 50.5715) (14.444, 50.7956) knots 0 0 0 1 2 2 2
  spline S213 degree 2 poles (14.444, 50.7956) (14.444, 50.9201) (14.6482, 51.1143) (14.8075, 51.1143) knots 0 0 0 1 2 2 2
  spline S214 degree 2 poles (14.8075, 51.1143) (14.9221, 51.1143) (15.1014, 51.0396) (15.3106, 50.8902) knots 0 0 0 1 2 2 2
  spline S215 degree 2 poles (15.3106, 50.8902) (15.6492, 50.6611) (15.9979, 50.6561) knots 0 0 0 1 1 1
  spline S216 degree 2 poles (15.9979, 50.6561) (16.5208, 50.6561) (17.3226, 51.453) (17.3226, 52.0257) knots 0 0 0 1 2 2 2
  spline S217 degree 2 poles (17.3226, 52.0257) (17.3226, 52.5786) (16.6104, 53.5398) (15.9829, 53.7988) knots 0 0 0 1 2 2 2
  spline S218 degree 2 poles (15.9829, 53.7988) (15.4948, 54.003) (14.6482, 54.0328) knots 0 0 0 1 1 1
  line L134 (14.6482, 54.0328) -> (15.8186, 56.3985)
  line L135 (15.8186, 56.3985) -> (18.005, 56.3985)
  spline S219 degree 2 poles (18.9463, 53.3157) (18.9463, 54.3566) (19.5738, 55.8606) (20.0967, 56.2292) knots 0 0 0 1 2 2 2
  spline S220 degree 2 poles (20.0967, 56.2292) (20.5001, 56.523) (20.9334, 56.523) knots 0 0 0 1 1 1
  spline S221 degree 2 poles (20.9334, 56.523) (21.6357, 56.523) (22.1935, 55.8108) knots 0 0 0 1 1 1
  spline S222 degree 2 poles (22.1935, 55.8108) (22.8907, 54.9243) (22.8907, 53.4103) knots 0 0 0 1 1 1
  spline S223 degree 2 poles (22.8907, 53.4103) (22.8907, 52.3495) (22.2781, 50.8653) (21.3319, 50.1979) (20.8886, 50.1979) knots 0 0 0 1 2 3 3 3
  spline S224 degree 2 poles (20.8886, 50.1979) (20.017, 50.1979) (19.4343, 51.2289) knots 0 0 0 1 1 1
  spline S225 degree 2 poles (19.4343, 51.2289) (18.9463, 52.0955) (18.9463, 53.3157) knots 0 0 0 1 1 1
  spline S226 degree 2 poles (19.8278, 53.2011) (19.8278, 51.9461) (20.1366, 51.1492) knots 0 0 0 1 1 1
  spline S227 degree 2 poles (20.1366, 51.1492) (20.3955, 50.4818) (20.9035, 50.4818) knots 0 0 0 1 1 1
  spline S228 degree 2 poles (20.9035, 50.4818) (21.1476, 50.4818) (21.6655, 50.9151) (21.8, 51.4281) knots 0 0 0 1 2 2 2
  spline S229 degree 2 poles (21.8, 51.4281) (22.0092, 52.2001) (22.0092, 53.6045) knots 0 0 0 1 1 1
  spline S230 degree 2 poles (22.0092, 53.6045) (22.0092, 54.6504) (21.795, 55.3427) knots 0 0 0 1 1 1
  spline S231 degree 2 poles (21.795, 55.3427) (21.6307, 55.8606) (21.3767, 56.0748) knots 0 0 0 1 1 1
  spline S232 degree 2 poles (21.3767, 56.0748) (21.1924, 56.2242) (20.9285, 56.2242) knots 0 0 0 1 1 1
  spline S233 degree 2 poles (20.9285, 56.2242) (20.6246, 56.2242) (20.3856, 55.9503) knots 0 0 0 1 1 1
  spline S234 degree 2 poles (20.3856, 55.9503) (20.0619, 55.5768) (19.8278, 53.9781) (19.8278, 53.2011) knots 0 0 0 1 2 2 2
  spline S235 degree 2 poles (23.5531, 53.3157) (23.5531, 54.3566) (24.1806, 55.8606) (24.7036, 56.2292) knots 0 0 0 1 2 2 2
  spline S236 degree 2 poles (24.7036, 56.2292) (25.107, 56.523) (25.5403, 56.523) knots 0 0 0 1 1 1
  spline S237 degree 2 poles (25.5403, 56.523) (26.2425, 56.523) (26.8003, 55.8108) knots 0 0 0 1 1 1
  spline S238 degree 2 poles (26.8003, 55.8108) (27.4976, 54.9243) (27.4976, 53.4103) knots 0 0 0 1 1 1
  spline S239 degree 2 poles (27.4976, 53.4103) (27.4976, 52.3495) (26.885, 50.8653) (25.9387, 50.1979) (25.4955, 50.1979) knots 0 0 0 1 2 3 3 3
  spline S240 degree 2 poles (25.4955, 50.1979) (24.6239, 50.1979) (24.0412, 51.2289) knots 0 0 0 1 1 1
  spline S241 degree 2 poles (24.0412, 51.2289) (23.5531, 52.0955) (23.5531, 53.3157) knots 0 0 0 1 1 1
  spline S242 degree 2 poles (24.4346, 53.2011) (24.4346, 51.9461) (24.7434, 51.1492) knots 0 0 0 1 1 1
  spline S243 degree 2 poles (24.7434, 51.1492) (25.0024, 50.4818) (25.5104, 50.4818) knots 0 0 0 1 1 1
  spline S244 degree 2 poles (25.5104, 50.4818) (25.7545, 50.4818) (26.2724, 50.9151) (26.4069, 51.4281) knots 0 0 0 1 2 2 2
  spline S245 degree 2 poles (26.4069, 51.4281) (26.6161, 52.2001) (26.6161, 53.6045) knots 0 0 0 1 1 1
  spline S246 degree 2 poles (26.6161, 53.6045) (26.6161, 54.6504) (26.4019, 55.3427) knots 0 0 0 1 1 1
  spline S247 degree 2 poles (26.4019, 55.3427) (26.2375, 55.8606) (25.9835, 56.0748) knots 0 0 0 1 1 1
  spline S248 degree 2 poles (25.9835, 56.0748) (25.7993, 56.2242) (25.5353, 56.2242) knots 0 0 0 1 1 1
  spline S249 degree 2 poles (25.5353, 56.2242) (25.2315, 56.2242) (24.9925, 55.9503) knots 0 0 0 1 1 1
  spline S250 degree 2 poles (24.9925, 55.9503) (24.6687, 55.5768) (24.4346, 53.9781) (24.4346, 53.2011) knots 0 0 0 1 2 2 2
  spline S251 degree 2 poles (28.16, 53.3157) (28.16, 54.3566) (28.7875, 55.8606) (29.3105, 56.2292) knots 0 0 0 1 2 2 2
  spline S252 degree 2 poles (29.3105, 56.2292) (29.7139, 56.523) (30.1472, 56.523) knots 0 0 0 1 1 1
  spline S253 degree 2 poles (30.1472, 56.523) (30.8494, 56.523) (31.4072, 55.8108) knots 0 0 0 1 1 1
  spline S254 degree 2 poles (31.4072, 55.8108) (32.1045, 54.9243) (32.1045, 53.4103) knots 0 0 0 1 1 1
  spline S255 degree 2 poles (32.1045, 53.4103) (32.1045, 52.3495) (31.4919, 50.8653) (30.5456, 50.1979) (30.1023, 50.1979) knots 0 0 0 1 2 3 3 3
  spline S256 degree 2 poles (30.1023, 50.1979) (29.2308, 50.1979) (28.6481, 51.2289) knots 0 0 0 1 1 1
  spline S257 degree 2 poles (28.6481, 51.2289) (28.16, 52.0955) (28.16, 53.3157) knots 0 0 0 1 1 1
  spline S258 degree 2 poles (29.0415, 53.2011) (29.0415, 51.9461) (29.3503, 51.1492) knots 0 0 0 1 1 1
  spline S259 degree 2 poles (29.3503, 51.1492) (29.6093, 50.4818) (30.1173, 50.4818) knots 0 0 0 1 1 1
  spline S260 degree 2 poles (30.1173, 50.4818) (30.3613, 50.4818) (30.8793, 50.9151) (31.0137, 51.4281) knots 0 0 0 1 2 2 2
  spline S261 degree 2 poles (31.0137, 51.4281) (31.2229, 52.2001) (31.2229, 53.6045) knots 0 0 0 1 1 1
  spline S262 degree 2 poles (31.2229, 53.6045) (31.2229, 54.6504) (31.0088, 55.3427) knots 0 0 0 1 1 1
  spline S263 degree 2 poles (31.0088, 55.3427) (30.8444, 55.8606) (30.5904, 56.0748) knots 0 0 0 1 1 1
  spline S264 degree 2 poles (30.5904, 56.0748) (30.4061, 56.2242) (30.1422, 56.2242) knots 0 0 0 1 1 1
  spline S265 degree 2 poles (30.1422, 56.2242) (29.8384, 56.2242) (29.5993, 55.9503) knots 0 0 0 1 1 1
  spline S266 degree 2 poles (29.5993, 55.9503) (29.2756, 55.5768) (29.0415, 53.9781) (29.0415, 53.2011) knots 0 0 0 1 2 2 2
  spline S267 degree 2 poles (32.7668, 53.3157) (32.7668, 54.3566) (33.3944, 55.8606) (33.9173, 56.2292) knots 0 0 0 1 2 2 2
  spline S268 degree 2 poles (33.9173, 56.2292) (34.3207, 56.523) (34.754, 56.523) knots 0 0 0 1 1 1
  spline S269 degree 2 poles (34.754, 56.523) (35.4563, 56.523) (36.0141, 55.8108) knots 0 0 0 1 1 1
  spline S270 degree 2 poles (36.0141, 55.8108) (36.7113, 54.9243) (36.7113, 53.4103) knots 0 0 0 1 1 1
  spline S271 degree 2 poles (36.7113, 53.4103) (36.7113, 52.3495) (36.0987, 50.8653) (35.1525, 50.1979) (34.7092, 50.1979) knots 0 0 0 1 2 3 3 3
  spline S272 degree 2 poles (34.7092, 50.1979) (33.8376, 50.1979) (33.2549, 51.2289) knots 0 0 0 1 1 1
  spline S273 degree 2 poles (33.2549, 51.2289) (32.7668, 52.0955) (32.7668, 53.3157) knots 0 0 0 1 1 1
  spline S274 degree 2 poles (33.6484, 53.2011) (33.6484, 51.9461) (33.9572, 51.1492) knots 0 0 0 1 1 1
  spline S275 degree 2 poles (33.9572, 51.1492) (34.2161, 50.4818) (34.7241, 50.4818) knots 0 0 0 1 1 1
  spline S276 degree 2 poles (34.7241, 50.4818) (34.9682, 50.4818) (35.4861, 50.9151) (35.6206, 51.4281) knots 0 0 0 1 2 2 2
  spline S277 degree 2 poles (35.6206, 51.4281) (35.8298, 52.2001) (35.8298, 53.6045) knots 0 0 0 1 1 1
  spline S278 degree 2 poles (35.8298, 53.6045) (35.8298, 54.6504) (35.6156, 55.3427) knots 0 0 0 1 1 1
  spline S279 degree 2 poles (35.6156, 55.3427) (35.4513, 55.8606) (35.1973, 56.0748) knots 0 0 0 1 1 1
  spline S280 degree 2 poles (35.1973, 56.0748) (35.013, 56.2242) (34.749, 56.2242) knots 0 0 0 1 1 1
  spline S281 degree 2 poles (34.749, 56.2242) (34.4452, 56.2242) (34.2062, 55.9503) knots 0 0 0 1 1 1
  spline S282 degree 2 poles (34.2062, 55.9503) (33.8825, 55.5768) (33.6484, 53.9781) (33.6484, 53.2011) knots 0 0 0 1 2 2 2
  line L136 (38.1158, 55.8009) -> (39.5999, 56.523)
  line L137 (39.5999, 56.523) -> (39.7494, 56.523)
  line L138 (39.7494, 56.523) -> (39.7494, 51.3783)
  spline S283 degree 2 poles (39.7494, 51.3783) (39.7494, 50.8653) (39.834, 50.6113) (40.103, 50.4768) (40.5163, 50.4669) knots 0 0 0 1 2 3 3 3
  line L139 (40.5163, 50.4669) -> (40.5163, 50.3025)
  line L140 (40.5163, 50.3025) -> (38.2254, 50.3025)
  line L141 (38.2254, 50.3025) -> (38.2254, 50.4669)
  spline S284 degree 2 poles (38.2254, 50.4669) (38.6586, 50.4768) (38.9077, 50.6063) (39.0073, 50.8255) (39.0073, 51.3783) knots 0 0 0 1 2 3 3 3
  line L142 (39.0073, 51.3783) -> (39.0073, 54.6653)
  spline S285 degree 2 poles (39.0073, 54.6653) (39.0073, 55.3327) (38.9625, 55.522) knots 0 0 0 1 1 1
  spline S286 degree 2 poles (38.9625, 55.522) (38.9326, 55.6664) (38.7632, 55.8009) (38.6487, 55.8009) knots 0 0 0 1 2 2 2
  spline S287 degree 2 poles (38.6487, 55.8009) (38.4794, 55.8009) (38.1855, 55.6614) knots 0 0 0 1 1 1
  line L143 (38.1855, 55.6614) -> (38.1158, 55.8009)
  line L144 (-21.1658, 41.8312) -> (-21.5941, 40.6608)
  line L145 (-21.5941, 40.6608) -> (-25.19, 40.6608)
  line L146 (-25.19, 40.6608) -> (-25.19, 40.8252)
  spline S288 degree 2 poles (-25.19, 40.8252) (-23.6012, 42.2745) (-22.3063, 44.1073) (-22.3063, 44.8693) knots 0 0 0 1 2 2 2
  spline S289 degree 2 poles (-22.3063, 44.8693) (-22.3063, 45.447) (-23.0185, 46.194) (-23.5116, 46.194) knots 0 0 0 1 2 2 2
  spline S290 degree 2 poles (-23.5116, 46.194) (-23.9648, 46.194) (-24.677, 45.6661) (-24.8513, 45.1581) knots 0 0 0 1 2 2 2
  line L147 (-24.8513, 45.1581) -> (-25.0157, 45.1581)
  spline S291 degree 2 poles (-25.0157, 45.1581) (-24.9011, 45.9898) (-23.9748, 46.8813) (-23.2775, 46.8813) knots 0 0 0 1 2 2 2
  spline S292 degree 2 poles (-23.2775, 46.8813) (-22.5354, 46.8813) (-21.5394, 45.9301) (-21.5394, 45.2826) knots 0 0 0 1 2 2 2
  spline S293 degree 2 poles (-21.5394, 45.2826) (-21.5394, 44.8195) (-21.7535, 44.3563) knots 0 0 0 1 1 1
  spline S294 degree 2 poles (-21.7535, 44.3563) (-22.0872, 43.6291) (-22.8343, 42.8124) knots 0 0 0 1 1 1
  spline S295 degree 2 poles (-22.8343, 42.8124) (-23.9548, 41.5922) (-24.2337, 41.3382) knots 0 0 0 1 1 1
  line L148 (-24.2337, 41.3382) -> (-22.64, 41.3382)
  spline S296 degree 2 poles (-22.64, 41.3382) (-22.1519, 41.3382) (-21.7635, 41.4079) (-21.4497, 41.632) (-21.3302, 41.8312) knots 0 0 0 1 2 3 3 3
  line L149 (-21.3302, 41.8312) -> (-21.1658, 41.8312)
  line L150 (-20.2992, 40.5363) -> (-20.2992, 40.7007)
  spline S297 degree 2 poles (-20.2992, 40.7007) (-19.7115, 40.7106) (-18.7055, 41.2336) (-17.7642, 42.5484) (-17.575, 43.3353) knots 0 0 0 1 2 3 3 3
  spline S298 degree 2 poles (-17.575, 43.3353) (-18.2822, 42.8821) (-18.8549, 42.8821) knots 0 0 0 1 1 1
  spline S299 degree 2 poles (-18.8549, 42.8821) (-19.5024, 42.8821) (-20.4188, 43.8732) (-20.4188, 44.6999) knots 0 0 0 1 2 2 2
  spline S300 degree 2 poles (-20.4188, 44.6999) (-20.4188, 45.4968) (-19.9606, 46.1243) knots 0 0 0 1 1 1
  spline S301 degree 2 poles (-19.9606, 46.1243) (-19.4077, 46.8813) (-18.5163, 46.8813) knots 0 0 0 1 1 1
  spline S302 degree 2 poles (-18.5163, 46.8813) (-17.7642, 46.8813) (-17.2263, 46.2588) knots 0 0 0 1 1 1
  spline S303 degree 2 poles (-17.2263, 46.2588) (-16.5689, 45.4918) (-16.5689, 44.3662) knots 0 0 0 1 1 1
  spline S304 degree 2 poles (-16.5689, 44.3662) (-16.5689, 43.3502) (-17.57, 41.5922) (-18.4615, 41.0144) knots 0 0 0 1 2 2 2
  spline S305 degree 2 poles (-18.4615, 41.0144) (-19.1886, 40.5363) (-20.0403, 40.5363) knots 0 0 0 1 1 1
  line L151 (-20.0403, 40.5363) -> (-20.2992, 40.5363)
  spline S306 degree 2 poles (-17.5052, 43.669) (-17.4255, 44.2517) (-17.4255, 44.6003) knots 0 0 0 1 1 1
  spline S307 degree 2 poles (-17.4255, 44.6003) (-17.4255, 45.0386) (-17.7244, 46.0496) (-18.2672, 46.5875) (-18.6159, 46.5875) knots 0 0 0 1 2 3 3 3
  spline S308 degree 2 poles (-18.6159, 46.5875) (-19.0143, 46.5875) (-19.6169, 45.8703) (-19.6169, 45.1581) knots 0 0 0 1 2 2 2
  spline S309 degree 2 poles (-19.6169, 45.1581) (-19.6169, 44.2118) (-19.2185, 43.6789) knots 0 0 0 1 1 1
  spline S310 degree 2 poles (-19.2185, 43.6789) (-18.9246, 43.2905) (-18.4963, 43.2905) knots 0 0 0 1 1 1
  spline S311 degree 2 poles (-18.4963, 43.2905) (-18.2872, 43.2905) (-17.7194, 43.4897) (-17.5052, 43.669) knots 0 0 0 1 2 2 2
  line L152 (-14.6863, 46.1343) -> (-14.6863, 44.7796)
  line L153 (-14.6863, 44.7796) -> (-13.7251, 44.7796)
  line L154 (-13.7251, 44.7796) -> (-13.7251, 44.4658)
  line L155 (-13.7251, 44.4658) -> (-14.6863, 44.4658)
  line L156 (-14.6863, 44.4658) -> (-14.6863, 41.7914)
  spline S312 degree 2 poles (-14.6863, 41.7914) (-14.6863, 41.3929) (-14.4572, 41.114) (-14.2779, 41.114) knots 0 0 0 1 2 2 2
  spline S313 degree 2 poles (-14.2779, 41.114) (-14.1285, 41.114) (-13.8446, 41.2983) (-13.7699, 41.4776) knots 0 0 0 1 2 2 2
  line L157 (-13.7699, 41.4776) -> (-13.5956, 41.4776)
  spline S314 degree 2 poles (-13.5956, 41.4776) (-13.755, 41.0344) (-14.3327, 40.5911) (-14.6365, 40.5911) knots 0 0 0 1 2 2 2
  spline S315 degree 2 poles (-14.6365, 40.5911) (-14.8457, 40.5911) (-15.2441, 40.8202) (-15.4334, 41.2485) (-15.4334, 41.6918) knots 0 0 0 1 2 3 3 3
  line L158 (-15.4334, 41.6918) -> (-15.4334, 44.4658)
  line L159 (-15.4334, 44.4658) -> (-16.0858, 44.4658)
  line L160 (-16.0858, 44.4658) -> (-16.0858, 44.6153)
  spline S316 degree 2 poles (-16.0858, 44.6153) (-15.8368, 44.7149) (-15.3188, 45.183) (-15.1146, 45.5068) knots 0 0 0 1 2 2 2
  spline S317 degree 2 poles (-15.1146, 45.5068) (-15.0101, 45.6811) (-14.8258, 46.1343) knots 0 0 0 1 1 1
  line L161 (-14.8258, 46.1343) -> (-14.6863, 46.1343)
  line L162 (-12.1165, 47.0557) -> (-12.1165, 44.0425)
  spline S318 degree 2 poles (-12.1165, 44.0425) (-11.6184, 44.5904) (-11.0357, 44.8991) (-10.7419, 44.8991) knots 0 0 0 1 2 2 2
  spline S319 degree 2 poles (-10.7419, 44.8991) (-10.3932, 44.8991) (-9.8852, 44.5107) (-9.7657, 44.0973) knots 0 0 0 1 2 2 2
  spline S320 degree 2 poles (-9.7657, 44.0973) (-9.681, 43.8134) (-9.681, 43.0464) knots 0 0 0 1 1 1
  line L163 (-9.681, 43.0464) -> (-9.681, 41.5922)
  spline S321 degree 2 poles (-9.681, 41.5922) (-9.681, 41.2037) (-9.6163, 41.0593) knots 0 0 0 1 1 1
  spline S322 degree 2 poles (-9.6163, 41.0593) (-9.5715, 40.9497) (-9.3573, 40.8252) (-9.0685, 40.8252) knots 0 0 0 1 2 2 2
  line L164 (-9.0685, 40.8252) -> (-9.0685, 40.6608)
  line L165 (-9.0685, 40.6608) -> (-11.0955, 40.6608)
  line L166 (-11.0955, 40.6608) -> (-11.0955, 40.8252)
  line L167 (-11.0955, 40.8252) -> (-11.0008, 40.8252)
  spline S323 degree 2 poles (-11.0008, 40.8252) (-10.712, 40.8252) (-10.4879, 40.9995) (-10.443, 41.1688) knots 0 0 0 1 2 2 2
  spline S324 degree 2 poles (-10.443, 41.1688) (-10.4281, 41.2435) (-10.4281, 41.5922) knots 0 0 0 1 1 1
  line L168 (-10.4281, 41.5922) -> (-10.4281, 43.0464)
  spline S325 degree 2 poles (-10.4281, 43.0464) (-10.4281, 43.7238) (-10.5675, 44.1471) (-10.8714, 44.3563) (-11.0905, 44.3563) knots 0 0 0 1 2 3 3 3
  spline S326 degree 2 poles (-11.0905, 44.3563) (-11.3096, 44.3563) (-11.7828, 44.1222) (-12.1165, 43.7686) knots 0 0 0 1 2 2 2
  line L169 (-12.1165, 43.7686) -> (-12.1165, 41.5922)
  spline S327 degree 2 poles (-12.1165, 41.5922) (-12.1165, 41.1688) (-12.0218, 40.9646) (-11.7628, 40.8252) (-11.4491, 40.8252) knots 0 0 0 1 2 3 3 3